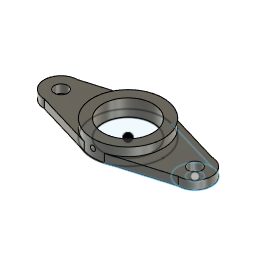
Component 3 (Autodesk Fusion 360 design; units mm, degrees)
Autodesk Fusion 360 part; units mm, degrees
note: some values were not read from the file. Set by a fixed rule: which sketch regions a step uses.
sketch "Sketch1" plane through (0, 0, 0) normal (0, 0, 1) x (1, 0, 0)
  circle A0 centre (0, 0) radius 15
  circle A1 centre (0, 0) radius 21
  circle A2 centre (40, 0) radius 10
  circle A3 centre (40, 0) radius 4
  line L0 (5.9934, 20.1266) -> (40, 10)
  line L1 (5.9934, -20.1266) -> (40, -10)
  dimension "d1" = 30
  dimension "d2" = 42
  dimension "d3" = 20
  dimension "d4" = 8
  dimension "d5" = 40
  constraint coincident A0.centre A1.centre
  constraint concentric A0 A1
  constraint concentric A2 A3
  constraint coincident A1 L0.start
  constraint tangent A1 L0
  constraint coincident A2 L0.end
  constraint coincident A1 L1.start
  constraint tangent A1 L1
  constraint coincident A2 L1.end
  measures "d1" diameter of A0
  measures "d2" diameter of A1
  measures "d3" diameter of A2
  measures "d4" diameter of A3
  measures "d5" distance of A0.centre A2.centre
extrude "Extrude1" add sketch "Sketch1" along normal blind 5 contours A1 A2 L0 L1 makes body 1
extrude "Extrude2" add sketch "Sketch1" along normal blind 5 contours A2 bodies 1
extrude "Extrude3" add sketch "Sketch1" along normal blind 10 contours A1 bodies 1
pattern_circular "C-Pattern1" count 2 over 360 about axis through (0, 0, 1.75) along (0, 0, 1) of "Extrude1", "Extrude2", "Extrude3" makes body 2
sketch "Sketch2" plane through (0, 0, 0) normal (0, 1, 0) x (1, 0, 0)
  line L0 (-21, 0) -> (21, -10)
  circle A0 centre (0, -5) radius 1.5
  dimension "d14" = 3
  constraint midpoint L0 A0.centre
  measures "d14" diameter of A0
extrude "Extrude4" cut sketch "Sketch2" against normal blind 41 bodies 1 2
